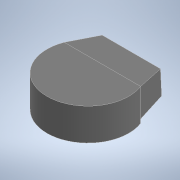
# Autodesk Inventor part: vez
Saved by Autodesk Inventor 2022 (Build 260153000, 153)
## iProperties
Created: 2022-11-29
Part Number: vez
Material: Generic
Document SubType Name: Modeling
Designer: matys
Density: 1 g/cm^3
Appearance: Gray
Author: matys
Autodesk Inventor part; units mm, degrees
ref_plane "YZ Plane" through (0, 0, 0) normal (1, 0, 0) x (0, 1, 0)
ref_plane "XZ Plane" through (0, 0, 0) normal (0, 1, 0) x (-1, 0, 0)
ref_plane "XY Plane" through (0, 0, 0) normal (0, 0, 1) x (1, 0, 0)
sketch "Sketch1" plane through (0, 0, 0) normal (0, 1, 0) x (-1, 0, 0)
  arc A0 (40.6448, -15.5) -> (-40.6448, -15.5) centre (0, 0) ccw
  line L0 (0, 0) -> (0, -48)
  line L1 (0, -48) -> (30.5, -48)
  line L2 (0, -48) -> (-30.5, -48)
  line L3 (0, 43.5) -> (0, -15.5)
  line L4 (0, -15.5) -> (40.6448, -15.5)
  line L5 (30.5, -48) -> (40.6448, -15.5)
  line L6 (0, -15.5) -> (-40.6448, -15.5)
  line L7 (-30.5, -48) -> (-40.6448, -15.5)
  line L8 (43.5, 0) -> (41.5, 0)
  arc A1 (38.4968, -15.5) -> (-38.4968, -15.5) centre (0, 0) ccw
  line L9 (30.5, -48) -> (28.5, -48)
  line L10 (28.5, -48) -> (38.4968, -15.5)
  line L11 (-30.5, -48) -> (-40.6448, -15.5)
  line L12 (-28.5, -48) -> (-38.4968, -15.5)
  dimension "d0" = 87
  dimension "d1" = 48
  dimension "d2" = 30.5
  dimension "d3" = 30.5
  dimension "d4" = 59
  dimension "d5" = 2
  dimension "d6" = 2
  constraints: 26 end point, 7 point on circle, 4 point on line, 3 horizontal, 2 centre point, 2 coincident, 2 symmetric about line, 1 perpendicular, 1 vertical
  measures "d0" diameter of A0
  measures "d1" distance of L0.start L0.end
  measures "d2" distance of L0.end L1.end
  measures "d3" distance of L0.end L2.end
  measures "d4" distance of L3.start L3.end
  measures "d5" distance of L8.start L8.end
  measures "d6" distance of L1.end L9.end
extrude "Extrusion1" add sketch "Sketch1" along normal blind 30
chamfer "Chamfer1" distance 2 distance2 30 2 edges at (-15.25, 30, -48) (15.25, 30, -48) measured on face at (15.25, 30, -47.5) measured on face at (-15.25, 30, -47.5)
chamfer "Chamfer2" distance 4 distance2 30.5 2 edges at (-15.5621, 30, -46.0001) (15.5621, 30, -46.0001) measured on face at (-15.5621, 29.5011, -46.0334) measured on face at (15.5621, 29.5011, -46.0334)
sketch "Sketch2" plane through (0, 0, 0) normal (0, -1, 0) x (1, 0, 0)
  arc A0 (40.6448, -15.5) -> (-40.6448, -15.5) centre (0, 0) ccw projected
  line L0 (0, 43.5) -> (0, 41.5)
  line L1 (0, 43.5) -> (0, -15.5)
  line L2 (-40.6448, -15.5) -> (40.6448, -15.5) projected
  line L3 (0, -15.5) -> (40.6448, -15.5)
  line L4 (40.6448, -15.5) -> (-40.6448, -15.5)
  arc A1 (40.6448, -15.5) -> (-40.6448, -15.5) centre (0, 0) ccw
  line L5 (0, 0) -> (0, 30)
  circle A2 centre (0, 0) radius 30
  circle A3 centre (0, 0) radius 32
  line L6 (0, -32) -> (0, -36)
  line L7 (30.5, -48) -> (-30.5, -48) projected
  line L8 (0, -48) -> (30.5, -48)
  line L9 (30.5, -48) -> (15.25, -48)
  line L10 (15.25, -36) -> (0, -36)
  line L11 (15.25, -36) -> (40.6448, -15.5)
  line L12 (-15.25, -36) -> (-40.6448, -15.5)
  line L13 (-15.25, -36) -> (0, -36)
  circle A4 centre (0, 0) radius 32.5
  point P0 (-40.6448, -15.5)
  dimension "d18" = 64
  dimension "d15" = 2
  dimension "d16" = 59
  dimension "d17" = 30
  dimension "d19" = 4
  dimension "d24" = 65
  constraints: 24 end point, 3 coincident, 3 point on circle, 3 vertical, 2 centre point, 2 vertical alignment, 1 collinear, 1 midpoint, 1 parallel, 1 perpendicular, 1 point on line, 1 symmetric about line, 4 other
  measures "d15" distance of L0.start L0.end
  measures "d16" distance of L0.start L1.end
  measures "d17" distance of L5.start L5.end
  measures "d19" distance of L6.start L6.end
  measures "d24" diameter of A4
extrude "Extrusion2" add sketch "Sketch2" along normal blind 4
sketch "Sketch3" plane through (0, -4, 0) normal (0, -1, 0) x (1, 0, 0)
  line L0 (0, 0) -> (0, 30)
  circle A0 centre (0, 0) radius 30
  line L1 (0, 30) -> (0, 32.5)
  circle A1 centre (0, 0) radius 32.5
  dimension "d22" = 30
  dimension "d25" = 2.5
  constraints: 4 end point, 2 coincident, 2 point on circle, 2 vertical, 1 centre point, 1 vertical alignment, 2 other
  measures "d22" distance of L0.start L0.end
  measures "d25" distance of L1.start L1.end
extrude "Extrusion3" add sketch "Sketch3" along normal blind 5
sketch "Sketch4" plane through (0, -9, 0) normal (0, -1, 0) x (1, 0, 0)
  circle A0 centre (0, 0) radius 32.5 projected
  line L0 (0, 32.5) -> (0, 37.5)
  circle A1 centre (0, 0) radius 37.5
  circle A2 centre (0, 0) radius 30 projected
  line L1 (0, 30) -> (0, 26.5)
  circle A3 centre (0, 0) radius 26.5
  dimension "d28" = 5
  dimension "d29" = 3.5
  constraints: 4 end point, 4 vertical alignment, 2 coincident, 2 vertical, 6 other
  measures "d28" distance of L0.start L0.end
  measures "d29" distance of L1.start L1.end
extrude "Extrusion4" add sketch "Sketch4" along normal blind 5 contours A0 | A1 | A2
sketch "Sketch5" plane through (0, -4, 0) normal (0, -1, 0) x (1, 0, 0)
  circle A0 centre (0, 0) radius 30 projected
  line L0 (0, 30) -> (0, 26.5)
  circle A1 centre (0, 0) radius 26.5 projected
  circle A2 centre (0, 0) radius 30
  circle A3 centre (0, 0) radius 32.5
  constraints: 2 centre point, 2 coincident, 2 end point, 2 vertical alignment, 1 vertical, 3 other
extrude "Extrusion5" cut sketch "Sketch5" against normal blind 30 contours A0 | A1
sketch "Sketch6" plane through (0, -14, 0) normal (0, -1, 0) x (1, 0, 0)
  circle A0 centre (0, 0) radius 37.5
  constraints: 1 centre point, 1 coincident
extrude "Extrusion6" cut sketch "Sketch6" against normal blind 10
sketch "Sketch7" plane through (0, -4, 0) normal (0, -1, 0) x (1, 0, 0)
  circle A0 centre (0, 0) radius 30
  circle A1 centre (0, 0) radius 30 projected
  line L0 (0, -30) -> (0, -32.5)
  line L1 (15.25, -36) -> (-15.25, -36) projected
  circle A2 centre (0, 0) radius 32.5
  line L2 (30, 0) -> (33.5, 0)
  circle A3 centre (0, 0) radius 33.5
  dimension "d36" = 2.5
  dimension "d44" = 3.5
  constraints: 4 end point, 3 coincident, 2 point on circle, 1 centre point, 1 horizontal, 1 horizontal alignment, 1 perpendicular, 1 vertical alignment, 4 other
  measures "d36" distance of L0.start L0.end
  measures "d44" distance of L2.start L2.end
extrude "Extrusion7" cut sketch "Sketch7" against normal blind 5 contours L2 A2 L0 A0 | A0 L0 A2 L2 | A3
sketch "Sketch8" plane through (0, 1, 0) normal (0, -1, 0) x (1, 0, 0)
  circle A0 centre (0, 0) radius 30
  line L0 (32.5, 0) -> (-32.5, 0)
  line L1 (33.3654, -3) -> (-33.3654, -3)
  line L2 (33.3654, 3) -> (-33.3654, 3)
  line L3 (30, 0) -> (33.5, 0)
  circle A1 centre (0, 0) radius 33.5
  circle A2 centre (0, 0) radius 33.5 projected
  circle A3 centre (0, 0) radius 33.5
  point P0 (-29.8496, -3)
  point P1 (-29.8496, 3)
  point P2 (29.8496, 3)
  point P3 (29.8496, -3)
  dimension "d39" = 3
  dimension "d40" = 3
  dimension "d43" = 3.5
  constraints: 8 end point, 4 point on circle, 3 coincident, 2 horizontal, 2 parallel, 1 centre point, 1 horizontal alignment, 1 point on line, 6 other
  measures "d39" distance between parallel lines of L0 L1
  measures "d40" distance between parallel lines of L0 L2
  measures "d43" distance of L3.start L3.end
extrude "Extrusion8" cut sketch "Sketch8" against normal blind 5 contours L0 L3 A1 L1 A0 | A0 L2 A1 L3 L0 | A0 L1 A1 L2
sketch "Sketch9" plane through (0, -4, 0) normal (0, -1, 0) x (1, 0, 0)
  point P0 (0, 0)
ref_plane "Work Plane1" through (-40.6448, 15, -15.5) normal (0, 0, -1) x (-1, 0, 0)
sketch "Sketch12" plane through (-40.6448, 15, -15.5) normal (0, 0, -1) x (-1, 0, 0)
  line L0 (-71.686, 11.0089) -> (-71.1448, -15) projected
  line L1 (-10.1448, -15) -> (-9.6036, 11.0089) projected
  line L2 (-71.1448, -15) -> (-10.1448, -15)
  line L3 (-10.1448, -15) -> (-10.1448, 11.0089)
  line L4 (-71.686, 11.0089) -> (-9.6036, 11.0089) projected
  line L5 (-81.2896, -15) -> (-71.1448, -15) projected
  line L6 (-71.1448, -15) -> (-71.1448, 11.0089)
  line L7 (-71.1448, -15) -> (-71.1448, 11.0089)
  line L8 (-71.1448, 11.0089) -> (-10.6448, 11.0089)
  line L9 (-10.6448, -9) -> (-10.6448, 11) projected
  line L10 (-71.1448, -15) -> (-10.1448, -15) projected
  line L11 (-71.1448, -15) -> (-68.1448, -15)
  line L12 (-68.1448, -15) -> (-68.1448, -12)
  line L13 (-68.1448, -12) -> (-71.1448, -12)
  line L14 (-10.1448, -15) -> (-10.1448, 11.0089)
  line L15 (-10.1448, 11.0089) -> (-10.1448, 8.0089)
  line L16 (-10.1448, 8.0089) -> (-13.1448, 8.0089)
  line L17 (-13.1448, 8.0089) -> (-68.1448, 8.0089)
  line L18 (-68.1448, 8.0089) -> (-68.1448, -12)
  line L19 (-68.1448, -12) -> (-13.1448, -12)
  line L20 (-13.1448, -12) -> (-13.1448, 8.0089)
  point P0 (-40.6448, -15)
  dimension "d47" = 3
  dimension "d48" = 3
  dimension "d49" = 3
  dimension "d50" = 3
  constraints: 30 end point, 7 point on line, 6 perpendicular, 4 equal length, 2 horizontal
  measures "d47" distance of L0.end L11.end
  measures "d48" distance of L11.end L12.end
  measures "d49" distance of L3.end L15.end
  measures "d50" distance of L15.end L16.end
extrude "Extrusion9" cut sketch "Sketch12" along normal blind 50 and the other way blind 10 contours L18 L17 L20 L19
sketch "Sketch13" plane through (27.5, 3, -11.9896) normal (-1, 0, 0) x (0, 0, 1)
  line L0 (-35.8104, 0) -> (-34.4765, 20.0089) projected
  line L1 (-35.8104, 0) -> (-34.4765, 20.0089)
  line L2 (-35.8104, 0) -> (-35.1435, 10.0044)
  line L3 (-35.1435, 10.0044) -> (-3.5104, 10.0044)
  line L4 (-3.5104, -3) -> (-3.5104, 27) projected
  line L5 (-35.1435, 10.0044) -> (-30.1435, 10.0044)
  line L6 (-30.1435, 10.0044) -> (-30.1435, 5.0044)
  line L7 (-30.1435, 5.0044) -> (-35.4769, 5.0022)
  line L8 (-30.1435, 10.0044) -> (-30.1435, 15.0044)
  line L9 (-30.1435, 15.0044) -> (-34.8101, 15.0044)
  line L10 (-30.1435, 10.0044) -> (-25.1435, 10.0044)
  line L11 (-30.1435, 10.0044) -> (-25.1435, 10.0044)
  line L12 (-25.1435, 10.0044) -> (-25.1435, 5.5044)
  circle A0 centre (-25.1435, 10.0044) radius 4.5
  point P0 (11.9896, -3)
  dimension "d55" = 5
  dimension "d56" = 5
  dimension "d57" = 5
  dimension "d58" = 5
  dimension "d59" = 4.5
  constraints: 22 end point, 5 point on line, 3 perpendicular, 2 collinear, 2 midpoint, 1 coincident, 1 horizontal, 1 vertical alignment, 2 other
  measures "d55" distance of L2.end L5.end
  measures "d56" distance of L5.end L6.end
  measures "d57" distance of L5.end L8.end
  measures "d58" distance of L5.end L10.end
  measures "d59" distance of L10.end L12.end
extrude "Extrusion10" cut sketch "Sketch13" along normal blind 57 and the other way blind 2 contours L3 A0 | L12 A0 L3 | L3 A0 L12
body "Solid1"
